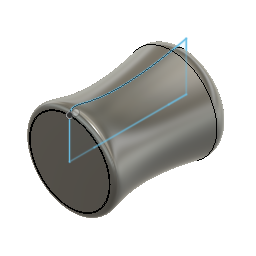
knob (Autodesk Fusion 360 design; units mm, degrees)
Autodesk Fusion 360 part; units mm, degrees
sketch "sketch 499" plane through (0, 0, 0) normal (1, 0, 0) x (0, 0, -1)
  line L0 (-9, -0.224) -> (-11.8934, -0.224)
  line L1 (-9, -0.224) -> (-9, 7.7499)
  spline S0 degree 5 poles (-9, 7.7499) (-9.6617, 7.5929) (-10.9648, 7.2988) (-12.8586, 6.9174) (-15.2596, 6.5305) (-18.0371, 6.2586) (-20.5611, 6.2025) (-22.7914, 6.3508) (-24.6824, 6.6616) (-26.1911, 7.0436) (-27.2896, 7.3339) (-27.8449, 7.2811) (-28.0872, 6.9661) (-28.1726, 6.6164) (-28.1964, 6.4066) knots 0 0 0 0 0 0 0.1 0.2 0.3 0.4 0.5 0.6 0.7 0.8 0.9 1 1 1 1 1 1
  arc A0 (-28.1964, 6.4066) -> (-28.2027, 6.2943) centre (-27.2027, 6.2943) ccw
  line L2 (-28.2027, 6.2943) -> (-28.2027, -0.224)
  line L3 (-24.157, -0.224) -> (-28.2027, -0.224)
  line L4 (-11.8934, -0.224) -> (-24.157, -0.224)
revolve "Revolve1" add sketch "sketch 499" angle 360 about axis through (0, -0.224, 9) along (0, 0, 1)
sketch "Sketch2" plane through (0, 0, 9) normal (0, 0, -1) x (-1, 0, 0)
  circle A0 centre (0, -0.224) radius 7.9739
  circle A1 centre (0, 0) radius 5.25
  dimension "d128" = 10.5
  constraint coincident A1.centre origin
  measures "d128" diameter of A1
extrude "Extrude3" cut sketch "Sketch2" against normal blind 2.5 contours A1
sketch "Sketch3" plane through (0, 0, 11.5) normal (0, 0, -1) x (-1, 0, 0)
  circle A0 centre (0, 0) radius 5.25
  circle A1 centre (0, 0) radius 2.5
  dimension "d131" = 5
  constraint coincident A0.centre A1.centre
  measures "d131" diameter of A1
extrude "Extrude4" cut sketch "Sketch3" against normal blind 6 contours A1
fillet "Fillet1" radius 2 1 edges at (-7.4343, 2.6595, 9)
